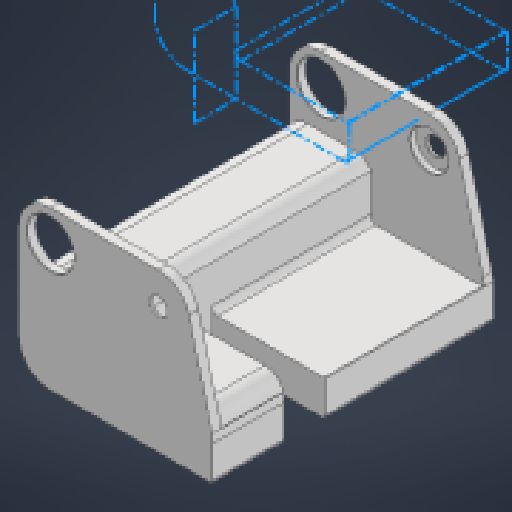
# Autodesk Inventor part: ServoMount
Saved by Autodesk Inventor 2024.1 (Build 281209000, 209)
## iProperties
Created: 2023-11-14
Part Number: ServoMount
Material: Generic
Document SubType Name: Modeling
Designer: Brandon
Density: 1 g/cm^3
Appearance: Default
Author: Brandon
Autodesk Inventor part; units mm, degrees
ref_plane "YZ Plane" through (0, 0, 0) normal (1, 0, 0) x (0, 1, 0)
ref_plane "XZ Plane" through (0, 0, 0) normal (0, 1, 0) x (-1, 0, 0)
ref_plane "XY Plane" through (0, 0, 0) normal (0, 0, 1) x (1, 0, 0)
sketch "Sketch1" plane through (0, 0, 0) normal (0, 0, 1) x (1, 0, 0)
  circle A0 centre (0, -4.5936) radius 3.81 projected
  circle A1 centre (0, -4.5936) radius 3.937
  arc A2 (0, 0.7404) -> (-5.334, -4.5936) centre (0, -4.5936) ccw
  line L0 (2.032, -6.6256) -> (-2.032, -6.6256) projected
  line L1 (2.032, -2.5616) -> (2.032, -6.6256) projected
  line L2 (-2.032, -2.5616) -> (2.032, -2.5616) projected
  line L3 (-2.032, -6.6256) -> (-2.032, -2.5616) projected
  circle A3 centre (18.288, -4.5936) radius 1.524
  arc A4 (23.4535, -3.2636) -> (18.288, 0.7404) centre (18.288, -4.5936) ccw
  line L4 (0, 0.7404) -> (18.288, 0.7404)
  line L5 (27.2953, -20.0494) -> (18.963, -20.0494) projected
  line L6 (18.963, -20.0494) -> (18.963, -25.2412) projected
  spline S0 degree 3 poles (18.963, -25.2412) (18.963, -25.3646) (18.9307, -25.4866) (18.8751, -25.5737) (18.8196, -25.6607) (18.7418, -25.7114) (18.663, -25.7114) knots 1.570796 1.570796 1.570796 1.570796 2.356194 2.356194 2.356194 3.141593 3.141593 3.141593 3.141593 projected
  line L7 (18.663, -25.7114) -> (17.913, -25.7114) projected
  spline S1 degree 3 poles (17.913, -25.7114) (17.8342, -25.7114) (17.7564, -25.6607) (17.7009, -25.5737) (17.6453, -25.4866) (17.613, -25.3646) (17.613, -25.2412) knots 0 0 0 0 0.785398 0.785398 0.785398 1.570796 1.570796 1.570796 1.570796 projected
  line L8 (17.613, -25.2412) -> (17.613, -20.0494) projected
  line L9 (17.613, -20.0494) -> (9.2807, -20.0494) projected
  arc A5 (8.988, -19.9974) -> (9.2807, -20.0494) centre (9.281, -19.1976) ccw projected
  line L10 (8.988, -19.9974) -> (8.988, -25.4082) projected
  arc A6 (8.988, -25.4082) -> (9.588, -26.0082) centre (9.588, -25.4082) ccw projected
  line L11 (9.588, -26.0082) -> (11.5899, -26.0082) projected
  arc A7 (14.9361, -26.0082) -> (11.5899, -26.0082) centre (13.263, -24.5414) ccw projected
  line L12 (14.9361, -26.0082) -> (21.6399, -26.0082) projected
  arc A8 (24.9861, -26.0082) -> (21.6399, -26.0082) centre (23.313, -24.5414) ccw projected
  line L13 (24.9861, -26.0082) -> (26.988, -26.0082) projected
  arc A9 (26.988, -26.0082) -> (27.588, -25.4082) centre (26.988, -25.4082) ccw projected
  line L14 (27.588, -25.4082) -> (27.588, -19.9974) projected
  arc A10 (27.2953, -20.0494) -> (27.588, -19.9974) centre (27.295, -19.1976) ccw projected
  arc A11 (-5.334, -20.6742) -> (0, -26.0082) centre (0, -20.6742) ccw
  line L15 (-5.334, -20.6742) -> (-5.334, -4.5936)
  line L16 (0, -26.0082) -> (26.988, -26.0082)
  arc A12 (27.588, -19.9974) -> (27.4195, -18.6675) centre (22.254, -19.9974) ccw
  line L17 (23.4535, -3.2636) -> (27.4195, -18.6675)
  circle A13 centre (0, -4.5936) radius 1.651 projected
  point P0 (0, 0)
  point P1 (-5.2119, -3.4587)
  dimension "d0" = 0.127
  dimension "d1" = 3.048
  dimension "d2" = 10.668
  dimension "d3" = 10.668
  dimension "d4" = 10.668
  constraints: 11 point on circle, 10 end point, 6 centre point, 6 tangent, 3 coincident, 2 horizontal, 1 vertical, 1 vertical alignment, 2 other
  measures "d0" radial gap between concentric circles of A0 A1
  measures "d1" diameter of A3
  measures "d2" diameter of A4
  measures "d3" diameter of A11
  measures "d4" diameter of A12
extrude "Extrusion1" add sketch "Sketch1" along normal blind 1.5875 contours L4 A4 L17 A12 A10 L5 L6 S0 L7 S1 L8 L9 A5 L10 A6 L16 A11 L15 A2 | A6 L10 A5 L9 L8 S1 L7 S0 L6 L5 A10 L14 A9 L13 A8 L12 A7 L11 | A7 L16 | A8 L16
sketch "Sketch2" plane through (0, 0, 0) normal (0, 0, -1) x (-1, 0, 0)
  circle A0 centre (-18.288, -4.5936) radius 1.524 projected
  circle A1 centre (-18.288, -4.5936) radius 3.175
  point P0 (0, 0)
  dimension "d7" = 6.35
  constraints: 1 centre point, 1 coincident
  measures "d7" diameter of A1
extrude "Extrusion2" cut sketch "Sketch2" against normal blind 1.0583
chamfer "Chamfer1" distance 0.127 angle 45 4 edges at (16.764, -4.5936, 1.0583) (21.463, -4.5936, 0) (-3.937, -4.5936, 0) (-3.937, -4.5936, 1.5875)
sketch "Sketch3" plane through (0, 0, 0) normal (0, 0, -1) x (-1, 0, 0)
  arc A0 (-9.2678, 7.377) -> (-8.8876, 8.9862) centre (-18.288, -20.2544) ccw projected
  line L0 (-8.8876, 8.9862) -> (-8.8876, -19.1925) projected
  spline S0 degree 3 poles (-8.8876, -19.1925) (-8.8876, -19.2975) (-8.9307, -19.4013) (-9.0047, -19.4753) (-9.0788, -19.5494) (-9.1825, -19.5925) (-9.2876, -19.5925) knots 2.356196 2.356196 2.356196 2.356196 3.141593 3.141593 3.141593 3.926989 3.926989 3.926989 3.926989 projected
  line L1 (-9.2876, -19.5925) -> (-27.2884, -19.5925) projected
  spline S1 degree 3 poles (-27.2884, -19.5925) (-27.3935, -19.5925) (-27.4972, -19.5494) (-27.5713, -19.4753) (-27.6453, -19.4013) (-27.6884, -19.2975) (-27.6884, -19.1925) knots 2.356196 2.356196 2.356196 2.356196 3.141593 3.141593 3.141593 3.926989 3.926989 3.926989 3.926989 projected
  line L2 (-27.6884, -19.1925) -> (-27.6884, 8.9862) projected
  arc A1 (-27.6884, 8.9862) -> (-27.3082, 7.377) centre (-18.288, 10.3579) ccw projected
  arc A2 (-27.288, 7.2515) -> (-27.3082, 7.377) centre (-27.688, 7.2515) ccw projected
  line L3 (-27.288, 7.2515) -> (-27.288, -13.4921) projected
  arc A3 (-27.288, -13.4921) -> (-26.888, -13.8921) centre (-26.888, -13.4921) ccw projected
  line L4 (-26.888, -13.8921) -> (-22.988, -13.8921) projected
  arc A4 (-22.6721, -14.0466) -> (-22.988, -13.8921) centre (-22.988, -14.2921) ccw projected
  arc A5 (-22.6721, -14.0466) -> (-13.9039, -14.0466) centre (-18.288, -10.6399) ccw projected
  arc A6 (-13.588, -13.8921) -> (-13.9039, -14.0466) centre (-13.588, -14.2921) ccw projected
  line L5 (-13.588, -13.8921) -> (-9.688, -13.8921) projected
  arc A7 (-9.688, -13.8921) -> (-9.288, -13.4921) centre (-9.688, -13.4921) ccw projected
  line L6 (-9.288, -13.4921) -> (-9.288, 7.2515) projected
  arc A8 (-9.2678, 7.377) -> (-9.288, 7.2515) centre (-8.888, 7.2515) ccw projected
  circle A9 centre (-18.288, -4.5936) radius 3.302 projected
  line L7 (-27.588, -25.4082) -> (-27.588, -19.9974) projected
  arc A10 (-27.588, -25.4082) -> (-26.988, -26.0082) centre (-26.988, -25.4082) ccw projected
  line L8 (0, -26.0082) -> (-26.988, -26.0082) projected
  arc A11 (0, -26.0082) -> (5.334, -20.6742) centre (0, -20.6742) ccw projected
  line L9 (5.334, -4.5936) -> (5.334, -20.6742) projected
  arc A12 (5.334, -4.5936) -> (0, 0.7404) centre (0, -4.5936) ccw projected
  line L10 (-18.288, 0.7404) -> (0, 0.7404) projected
  arc A13 (-18.288, 0.7404) -> (-23.4535, -3.2636) centre (-18.288, -4.5936) ccw projected
  line L11 (-27.4195, -18.6675) -> (-23.4535, -3.2636) projected
  arc A14 (-27.4195, -18.6675) -> (-27.588, -19.9974) centre (-22.254, -19.9974) ccw projected
  circle A15 centre (0, -4.5936) radius 4.064 projected
  line L12 (-27.2953, -20.0494) -> (-18.963, -20.0494) projected
  line L13 (-18.963, -20.0494) -> (-18.963, -25.2412) projected
  spline S2 degree 3 poles (-18.963, -25.2412) (-18.963, -25.3646) (-18.9307, -25.4866) (-18.8751, -25.5737) (-18.8196, -25.6607) (-18.7418, -25.7114) (-18.663, -25.7114) knots 1.570796 1.570796 1.570796 1.570796 2.356194 2.356194 2.356194 3.141593 3.141593 3.141593 3.141593 projected
  line L14 (-18.663, -25.7114) -> (-17.913, -25.7114) projected
  spline S3 degree 3 poles (-17.913, -25.7114) (-17.8342, -25.7114) (-17.7564, -25.6607) (-17.7009, -25.5737) (-17.6453, -25.4866) (-17.613, -25.3646) (-17.613, -25.2412) knots 0 0 0 0 0.785398 0.785398 0.785398 1.570796 1.570796 1.570796 1.570796 projected
  line L15 (-17.613, -25.2412) -> (-17.613, -20.0494) projected
  line L16 (-17.613, -20.0494) -> (-9.2807, -20.0494) projected
  arc A16 (-9.2807, -20.0494) -> (-8.988, -19.9974) centre (-9.281, -19.1976) ccw projected
  line L17 (-8.988, -19.9974) -> (-8.988, -25.4082) projected
  arc A17 (-9.588, -26.0082) -> (-8.988, -25.4082) centre (-9.588, -25.4082) ccw projected
  line L18 (-9.588, -26.0082) -> (-11.5899, -26.0082) projected
  arc A18 (-11.5899, -26.0082) -> (-14.9361, -26.0082) centre (-13.263, -24.5414) ccw projected
  line L19 (-14.9361, -26.0082) -> (-21.6399, -26.0082) projected
  arc A19 (-21.6399, -26.0082) -> (-24.9861, -26.0082) centre (-23.313, -24.5414) ccw projected
  line L20 (-24.9861, -26.0082) -> (-26.988, -26.0082) projected
  arc A20 (-27.588, -25.4082) -> (-26.988, -26.0082) centre (-26.988, -25.4082) ccw projected
  line L21 (-27.588, -25.4082) -> (-27.588, -19.9974) projected
  arc A21 (-27.588, -19.9974) -> (-27.2953, -20.0494) centre (-27.295, -19.1976) ccw projected
  circle A22 centre (0, -4.5936) radius 5.334
  line L22 (-26.7822, -16.1921) -> (-8.8876, -16.1921)
  line L23 (-8.8876, -10.9436) -> (5.334, -10.9436)
  point P0 (0, 0)
  dimension "d16" = 6.35
  constraints: 4 end point, 4 point on line, 1 coincident, 1 horizontal alignment, 1 parallel, 1 perpendicular, 1 tangent, 6 other
  measures "d16" distance from line of A12.centre L23
extrude "Extrusion3" add sketch "Sketch3" along normal blind 10.414 contours L23 L9 A11 L8 A17 L17 A16 L16 L15 S3 L14 S2 L13 L12 A21 A14 S1 L1 S0 L0 | L0 S0 L1 S1 A14 L11 L22 | L8 A18 A19 A10 L7 A21 L12 L13 S2 L14 S3 L15 L16 A16 L17 A17 | L8 A18 | L8 A19
fillet "Fillet1" radius 3.175 4 edges at (26.7822, -16.1921, -5.207) (8.8876, -16.1921, -5.207) (8.8876, -10.9436, -5.207) (-5.334, -10.9436, -5.207)
sketch "Sketch4" plane through (0, 0, -10.414) normal (0, 0, -1) x (-1, 0, 0)
  line L0 (-8.6395, -19.2082) -> (-8.6395, 19.7241) projected
  arc A0 (5.334, -14.1186) -> (2.159, -10.9436) centre (2.159, -14.1186) ccw projected
  line L1 (2.159, -10.9436) -> (-5.8088, -10.9436) projected
  arc A1 (-5.8088, -10.9436) -> (-8.9357, -13.5678) centre (-5.8088, -14.1186) ccw projected
  arc A2 (-12.0626, -16.1921) -> (-8.9357, -13.5678) centre (-12.0626, -13.0171) ccw projected
  line L2 (-12.0626, -16.1921) -> (-24.3211, -16.1921) projected
  arc A3 (-24.3211, -16.1921) -> (-27.3958, -18.5754) centre (-24.3211, -19.3671) ccw projected
  line L3 (-27.3958, -18.5754) -> (-27.4195, -18.6675) projected
  arc A4 (-27.4195, -18.6675) -> (-27.588, -19.9974) centre (-22.254, -19.9974) ccw projected
  line L4 (-27.588, -19.9974) -> (-27.588, -25.4082) projected
  arc A5 (-27.588, -25.4082) -> (-26.988, -26.0082) centre (-26.988, -25.4082) ccw projected
  line L5 (-26.988, -26.0082) -> (0, -26.0082) projected
  arc A6 (0, -26.0082) -> (5.334, -20.6742) centre (0, -20.6742) ccw projected
  line L6 (5.334, -20.6742) -> (5.334, -14.1186) projected
  line L7 (-8.5125, -12.454) -> (-8.5125, -26.0082)
  point P0 (0, 0)
  dimension "d17" = 0.127
  constraints: 2 end point, 1 parallel, 1 point on circle, 1 point on line
  measures "d17" distance between parallel lines of L0 L7
extrude "Extrusion4" add sketch "Sketch4" along normal blind 7.0104 contours L6 A6 L5 L7 A1 L1 A0
sketch "Sketch5" plane through (0, 0, -17.4244) normal (0, 0, -1) x (-1, 0, 0)
  arc A0 (-9.2756, -20.0544) -> (-8.988, -20.0043) centre (-9.2759, -19.2027) ccw projected
  line L0 (-9.2756, -20.0544) -> (-27.3004, -20.0544) projected
  arc A1 (-27.588, -20.0043) -> (-27.3004, -20.0544) centre (-27.3001, -19.2027) ccw projected
  line L1 (-27.588, -20.0043) -> (-27.588, -25.4082) projected
  arc A2 (-27.588, -25.4082) -> (-26.988, -26.0082) centre (-26.988, -25.4082) ccw projected
  line L2 (-26.988, -26.0082) -> (-24.9861, -26.0082) projected
  arc A3 (-21.6399, -26.0082) -> (-24.9861, -26.0082) centre (-23.313, -24.5414) ccw projected
  line L3 (-21.6399, -26.0082) -> (-14.9361, -26.0082) projected
  arc A4 (-11.5899, -26.0082) -> (-14.9361, -26.0082) centre (-13.263, -24.5414) ccw projected
  line L4 (-11.5899, -26.0082) -> (-9.588, -26.0082) projected
  arc A5 (-9.588, -26.0082) -> (-8.988, -25.4082) centre (-9.588, -25.4082) ccw projected
  line L5 (-8.988, -25.4082) -> (-8.988, -20.0043) projected
  arc A6 (-5.8088, -10.9436) -> (-8.5125, -12.454) centre (-5.8088, -14.1186) ccw projected
  line L6 (-8.5125, -12.454) -> (-8.5125, -26.0082) projected
  line L7 (-8.5125, -26.0082) -> (0, -26.0082) projected
  arc A7 (0, -26.0082) -> (5.334, -20.6742) centre (0, -20.6742) ccw projected
  line L8 (5.334, -20.6742) -> (5.334, -14.1186) projected
  arc A8 (5.334, -14.1186) -> (2.159, -10.9436) centre (2.159, -14.1186) ccw projected
  line L9 (2.159, -10.9436) -> (-5.8088, -10.9436) projected
  line L10 (-8.5125, -26.0082) -> (-8.5125, -12.454) projected
  arc A9 (-8.5125, -12.454) -> (-8.9357, -13.5678) centre (-5.8088, -14.1186) ccw projected
  arc A10 (-12.0626, -16.1921) -> (-8.9357, -13.5678) centre (-12.0626, -13.0171) ccw projected
  line L11 (-12.0626, -16.1921) -> (-24.3211, -16.1921) projected
  arc A11 (-24.3211, -16.1921) -> (-27.3958, -18.5754) centre (-24.3211, -19.3671) ccw projected
  line L12 (-27.3958, -18.5754) -> (-27.4195, -18.6675) projected
  arc A12 (-27.4195, -18.6675) -> (-27.588, -19.9974) centre (-22.254, -19.9974) ccw projected
  line L13 (-27.588, -19.9974) -> (-27.588, -25.4082) projected
  arc A13 (-27.588, -25.4082) -> (-26.988, -26.0082) centre (-26.988, -25.4082) ccw projected
  line L14 (-26.988, -26.0082) -> (-8.5125, -26.0082) projected
  circle A14 centre (-9.2759, -19.2027) radius 0.8518
  arc A15 (-9.2756, -20.0544) -> (-8.988, -20.0043) centre (-9.2759, -19.2027) ccw projected
  line L15 (-9.2756, -20.0544) -> (-27.3004, -20.0544) projected
  arc A16 (-27.588, -20.0043) -> (-27.3004, -20.0544) centre (-27.3001, -19.2027) ccw projected
  line L16 (-27.588, -20.0043) -> (-27.588, -25.4082) projected
  arc A17 (-27.588, -25.4082) -> (-26.988, -26.0082) centre (-26.988, -25.4082) ccw projected
  line L17 (-26.988, -26.0082) -> (-24.9861, -26.0082) projected
  arc A18 (-21.6399, -26.0082) -> (-24.9861, -26.0082) centre (-23.313, -24.5414) ccw projected
  line L18 (-21.6399, -26.0082) -> (-14.9361, -26.0082) projected
  arc A19 (-11.5899, -26.0082) -> (-14.9361, -26.0082) centre (-13.263, -24.5414) ccw projected
  line L19 (-11.5899, -26.0082) -> (-9.588, -26.0082) projected
  arc A20 (-9.588, -26.0082) -> (-8.988, -25.4082) centre (-9.588, -25.4082) ccw projected
  line L20 (-8.988, -25.4082) -> (-8.988, -20.0043) projected
  point P0 (0, 0)
  point P1 (-8.5125, -18.8249)
  constraints: 1 coincident, 3 other
extrude "Extrusion5" add sketch "Sketch5" along normal blind 26.7843 contours A0 L5 A5 L4 A4 L3 A3 L2 A2 L1 A1 L0 | A14 L6 L14 A5 L5 | L6 A6 L9 A8 L8 A7 L7 A14 | L14 A4 | A3 L14
sketch "Sketch6" plane through (0, 0, -44.2087) normal (0, 0, -1) x (-1, 0, 0)
  circle A0 centre (-18.288, -4.5936) radius 1.524 projected
  line L0 (-27.588, -25.4082) -> (-27.588, -19.9974) projected
  arc A1 (-27.4195, -18.6675) -> (-27.588, -19.9974) centre (-22.254, -19.9974) ccw projected
  line L1 (-27.4195, -18.6675) -> (-23.4535, -3.2636) projected
  arc A2 (-18.288, 0.7404) -> (-23.4535, -3.2636) centre (-18.288, -4.5936) ccw projected
  line L2 (-18.288, 0.7404) -> (0, 0.7404) projected
  arc A3 (5.334, -4.5936) -> (0, 0.7404) centre (0, -4.5936) ccw projected
  line L3 (5.334, -4.5936) -> (5.334, -20.6742) projected
  arc A4 (0, -26.0082) -> (5.334, -20.6742) centre (0, -20.6742) ccw projected
  line L4 (0, -26.0082) -> (-26.988, -26.0082) projected
  arc A5 (-27.588, -25.4082) -> (-26.988, -26.0082) centre (-26.988, -25.4082) ccw projected
  circle A6 centre (0, -4.5936) radius 4.064 projected
  point P0 (0, 0)
extrude "Extrusion6" add sketch "Sketch6" along normal blind 1.5875
sketch "Sketch7" plane through (0, 0, -44.2087) normal (0, 0, 1) x (1, 0, 0)
  circle A0 centre (18.288, -4.5936) radius 3.175 projected
  point P0 (0, 0)
extrude "Extrusion7" cut sketch "Sketch7" against normal blind 1.0583
chamfer "Chamfer2" distance 0.127 angle 45 4 edges at (4.064, -4.5936, -44.2087) (4.064, -4.5936, -45.7962) (19.812, -4.5936, -45.267) (15.113, -4.5936, -44.2087)
body "Solid1"
